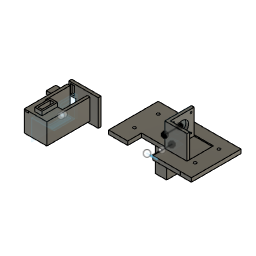
IgracZaBlututSviDelovi v9 (Autodesk Fusion 360 design; units mm, degrees)
Autodesk Fusion 360 part; units mm, degrees
note: some values were not read from the file. Chosen so that the rebuilt part matches the saved one: which bodies a step acts on. Set by a fixed rule: which sketch regions a step uses.
(part 1 of 2)
sketch "Sketch1" plane through (0, 0, 0) normal (0, 0, 1) x (1, 0, 0)
  line L0 (120.0463, 89.9645) -> (140.0463, 89.9645)
  line L1 (140.0463, -0.0355) -> (120.0463, -0.0355)
  line L2 (120.0463, -0.0355) -> (120.0463, 89.9645)
  line L3 (140.0463, 72.4645) -> (140.0463, 69.9645)
  circle A0 centre (140.0463, 69.9645) radius 2.5
  line L4 (140.0463, 69.9645) -> (140.0463, 67.4645)
  line L5 (140.0463, 32.4645) -> (140.0463, 29.9645)
  circle A1 centre (140.0463, 29.9645) radius 2.5
  line L6 (220.0463, 67.4645) -> (220.0463, 69.9645)
  line L7 (220.0463, 32.4645) -> (220.0463, 29.9645)
  circle A2 centre (220.0463, 69.9645) radius 2.5
  circle A3 centre (220.0463, 29.9645) radius 2.5
  line L8 (140.0463, 89.9645) -> (220, 89.9645)
  line L9 (220, 89.9645) -> (240, 89.9645)
  line L10 (240, 89.9645) -> (240, 40)
  line L11 (240, 40) -> (240, 0)
  line L12 (240, 0) -> (140, 0)
  line L13 (180.0463, 29.9645) -> (163.0463, 29.9645)
  line L14 (180.0463, 29.9645) -> (192.0463, 29.9645)
  line L15 (192.0463, 29.9645) -> (192.0463, 6.9645)
  line L16 (192.0463, 6.9645) -> (163.0463, 6.9645)
  line L17 (163.0463, 6.9645) -> (163.0463, 29.9645)
  line L18 (140.0463, 72.4645) -> (140.0463, 67.4645)
  line L19 (140.0463, 32.4645) -> (140.0463, 27.4645)
  line L20 (140.0463, 0) -> (140.0463, -0.0355)
  dimension "d1" = 20
  dimension "d2" = 90
  dimension "d3" = 20
  dimension "d4" = 5
  dimension "d8" = 5
  dimension "d17" = 5
  dimension "d18" = 5
  dimension "d21" = 17
  dimension "d22" = 12
  dimension "d23" = 23
  dimension "d24" = 29
  constraint horizontal L0
  constraint vertical L18
  constraint horizontal L1
  constraint vertical L2
  constraint perpendicular L0 L3
  constraint coincident L3.end A0.centre
  constraint parallel L4 L18
  constraint parallel L5 L18
  constraint coincident L5.end A1.centre
  constraint perpendicular L8 L18
  constraint perpendicular L9 L18
  constraint perpendicular L9 L10
  constraint perpendicular L12 L18
  constraint perpendicular L14 L15
  constraint perpendicular L15 L16
  constraint coincident A1 L5.start
  constraint collinear L18 L19
  constraint coincident A1 L19.end
  constraint coincident L12 L20.start
  constraint collinear L19 L20
  constraint coincident A3 L7.start
  constraint coincident A2 L6.start
  constraint coincident A0 L4.end
  constraint coincident A0 L3.start
  measures "d1" distance of L0.start L0.end
  measures "d2" distance of L0.start L1.end
  measures "d3" distance of L0.end L3.end
  measures "d4" diameter of A0
  measures "d8" diameter of A1
  measures "d17" diameter of A2
  measures "d18" diameter of A3
  measures "d21" distance of L13.start L13.end
  measures "d22" distance of L13.start L14.end
  measures "d23" distance of L14.end L15.end
  measures "d24" distance of L15.end L16.end
extrude "Extrude1" add sketch "Sketch1" along normal blind 7 makes body 1
sketch "Sketch2" plane through (0, 0, 7) normal (0, 0, 1) x (-1, 0, 0)
  circle A0 centre (-220.0463, -69.9645) radius 2.5
  line L0 (-163.0463, -29.9645) -> (-192.0463, -29.9645)
  line L1 (-192.0463, -29.9645) -> (-192.0463, -6.9645)
  line L2 (-192.0463, -6.9645) -> (-163.0463, -6.9645)
  line L3 (-163.0463, -6.9645) -> (-163.0463, -29.9645)
  circle A1 centre (-220.0463, -29.9645) radius 2.5
  circle A2 centre (-140.0463, -29.9645) radius 2.5
  circle A3 centre (-140.0463, -69.9645) radius 2.5
  line L4 (-140.0463, 0) -> (-240, 0)
  line L5 (-240, 0) -> (-240, -89.9645)
  line L6 (-240, -89.9645) -> (-120.0463, -89.9645)
  line L7 (-120.0463, -89.9645) -> (-120.0463, 0.0355)
  line L8 (-120.0463, 0.0355) -> (-140.0463, 0.0355)
  line L9 (-140.0463, 0.0355) -> (-140.0463, 0)
  line L10 (-163.0463, -29.9645) -> (-192.0463, -29.9645)
  line L11 (-192.0463, -29.9645) -> (-192.0463, -6.9645)
  line L12 (-192.0463, -6.9645) -> (-163.0463, -6.9645)
  line L13 (-163.0463, -6.9645) -> (-163.0463, -29.9645)
  constraint horizontal L10
  constraint vertical L11
  constraint horizontal L12
  constraint vertical L13
  constraint coincident L1.end L2.start
  constraint coincident L0.start L3.end
extrude "Extrude2" add sketch "Sketch2" against normal blind 4 contours L0 L1 L2 L3 L10 L11 L12 L13 bodies 1
extrude "Extrude3" add 1 faces at (172.7129, 14.6311, 3) along direction (0, 0, -1) blind 2 on bodies 1 bodies 1
extrude "Extrude4" cut 1 faces at (172.7129, 14.6311, 1) along direction (0, 0, 1) blind 50 on bodies 1 bodies 1
sketch "Sketch3" plane through (0, 0, 0) normal (0, 0, -1) x (1, 0, 0)
  circle A0 centre (220.0463, -69.9645) radius 2.5
  line L0 (192.0463, -29.9645) -> (163.0463, -29.9645)
  line L1 (163.0463, -29.9645) -> (163.0463, -6.9645)
  line L2 (163.0463, -6.9645) -> (192.0463, -6.9645)
  line L3 (192.0463, -6.9645) -> (192.0463, -29.9645)
  circle A1 centre (220.0463, -29.9645) radius 2.5
  circle A2 centre (140.0463, -29.9645) radius 2.5
  circle A3 centre (140.0463, -69.9645) radius 2.5
  line L4 (240, 0) -> (140.0463, 0)
  line L5 (140.0463, 0) -> (140.0463, 0.0355)
  line L6 (140.0463, 0.0355) -> (120.0463, 0.0355)
  line L7 (120.0463, 0.0355) -> (120.0463, -89.9645)
  line L8 (120.0463, -89.9645) -> (240, -89.9645)
  line L9 (240, -89.9645) -> (240, 0)
  line L10 (192.0463, -29.9645) -> (163.0463, -29.9645)
  line L11 (163.0463, -29.9645) -> (163.0463, -6.9645)
  line L12 (163.0463, -6.9645) -> (192.0463, -6.9645)
  line L13 (192.0463, -6.9645) -> (192.0463, -29.9645)
  constraint horizontal L10
  constraint vertical L11
  constraint horizontal L12
  constraint vertical L13
  constraint coincident L1.end L2.start
  constraint coincident L0.start L3.end
extrude "Extrude5" add sketch "Sketch3" against normal blind 4 contours L0 L1 L2 L3 L10 L11 L12 L13 bodies 1
sketch "Sketch4" plane through (0, 0, 0) normal (1, 0, 0) x (0, 1, 0)
sketch "Sketch5" plane through (0, 0, 7) normal (0, 0, 1) x (-1, 0, 0)
  line L0 (-163.0463, -6.9645) -> (-163.0463, -29.9645)
  line L1 (-163.0463, -29.9645) -> (-192.0463, -29.9645)
  line L2 (-192.0463, -29.9645) -> (-192.0463, -6.9645)
  line L3 (-192.0463, -6.9645) -> (-163.0463, -6.9645)
  circle A0 centre (-220.0463, -69.9645) radius 2.5
  circle A1 centre (-220.0463, -29.9645) radius 2.5
  circle A2 centre (-140.0463, -29.9645) radius 2.5
  circle A3 centre (-140.0463, -69.9645) radius 2.5
  line L4 (-140.0463, 0) -> (-240, 0)
  line L5 (-240, 0) -> (-240, -89.9645)
  line L6 (-240, -89.9645) -> (-120.0463, -89.9645)
  line L7 (-120.0463, -89.9645) -> (-120.0463, 0.0355)
  line L8 (-120.0463, 0.0355) -> (-140.0463, 0.0355)
  line L9 (-140.0463, 0.0355) -> (-140.0463, 0)
  line L10 (-50, -90) -> (-86, -90)
  line L11 (-86, -90) -> (-86, -30)
  line L12 (-86, -30) -> (-50, -30)
  line L13 (-50, -30) -> (-50, -90)
  dimension "d35" = 36
  dimension "d37" = 60
  constraint horizontal L10
  constraint vertical L11
  constraint horizontal L12
  constraint vertical L13
  measures "d35" distance of L10.start L10.end
  measures "d37" distance of L10.start L12.end
extrude "Extrude6" add sketch "Sketch5" along normal blind 7 separate body contours L10 L11 L12 L13 makes body 2
sketch "Sketch6" plane through (0, 0, 7) normal (0, 0, -1) x (1, 0, 0)
  line L0 (86, -30) -> (50, -30)
  line L1 (50, -30) -> (50, -90)
  line L2 (50, -90) -> (86, -90)
  line L3 (86, -90) -> (86, -30)
  line L4 (53.231, -87) -> (63, -87)
  line L5 (53.231, -87) -> (53, -87)
  line L6 (53, -87) -> (55, -87)
  line L7 (55, -87) -> (53, -87)
  line L8 (53, -87) -> (53, -78.5331)
  line L9 (53, -78.5331) -> (55, -78.5331)
  line L10 (55, -87) -> (58, -87)
  line L11 (58, -87) -> (63, -87)
  line L12 (63, -87) -> (58, -87)
  line L13 (58, -87) -> (58, -62)
  line L14 (58, -62) -> (63, -62)
  line L15 (63, -62) -> (63, -87)
  line L16 (58, -87) -> (53, -87)
  line L17 (53, -87) -> (53, -62)
  line L18 (53, -62) -> (58, -62)
  line L19 (58, -62) -> (58, -87)
  dimension "d42" = 2
  dimension "d43" = 3
  dimension "d44" = 5
  dimension "d45" = 25
  constraint perpendicular L3 L4
  constraint perpendicular L1 L5
  constraint horizontal L7
  constraint vertical L8
  constraint horizontal L9
  constraint parallel L4 L11
  constraint horizontal L12
  constraint vertical L13
  constraint horizontal L14
  constraint vertical L15
  constraint horizontal L16
  constraint vertical L17
  constraint horizontal L18
  constraint vertical L19
  measures "d42" distance of L6.end L5.end
  measures "d43" distance of L6.end L10.end
  measures "d44" distance of L10.end L4.end
  measures "d45" distance of L4.end L14.end
extrude "Extrude7" add sketch "Sketch6" along normal blind 7 contours L4 L5 L6 L7 L8 L10 L13 L16 L17 L18 L19 | L4 L11 L12 L13 L14 L15 L19 bodies 2
sketch "Sketch7" plane through (0, 0, 7) normal (0, 0, -1) x (1, 0, 0)
  line L0 (63, -62) -> (63, -87)
  line L1 (63, -87) -> (53, -87)
  line L2 (53, -87) -> (53, -62)
  line L3 (53, -62) -> (63, -62)
  line L4 (86, -30) -> (50, -30)
  line L5 (50, -30) -> (50, -90)
  line L6 (50, -90) -> (86, -90)
  line L7 (86, -90) -> (86, -30)
  line L8 (53, -87) -> (71, -87)
  line L9 (71, -87) -> (86, -87)
  line L10 (86, -87) -> (83, -87)
  line L11 (83, -87) -> (73, -87)
  line L12 (73, -87) -> (73, -62)
  line L13 (73, -62) -> (83, -62)
  line L14 (83, -62) -> (83, -87)
  dimension "d48" = 3
  dimension "d49" = 10
  dimension "d50" = 25
  constraint coincident L1.end L2.start
  constraint coincident L7 L9.end
  constraint perpendicular L7 L9
  constraint perpendicular L7 L10
  constraint horizontal L11
  constraint vertical L12
  constraint horizontal L13
  constraint vertical L14
  measures "d48" distance of L9.end L10.end
  measures "d49" distance of L10.end L11.end
  measures "d50" distance of L10.end L13.end
extrude "Extrude8" add sketch "Sketch7" along normal blind 7 contours L9 L11 L12 L13 L14 bodies 2
extrude "Extrude9" cut 1 faces at (59.6667, 75.8444, 0) along direction (0, 0, 1) blind 7 on bodies 2 bodies 2
sketch "Sketch8" plane through (73, 0, 0) normal (-1, 0, 0) x (0, -1, 0)
  line L0 (-62, 7) -> (-87, 7)
  line L1 (-87, 7) -> (-87, 0)
  line L2 (-87, 0) -> (-62, 0)
  line L3 (-62, 0) -> (-62, 7)
  line L4 (-87, 0) -> (-84.5, 0)
  line L5 (-84.5, 0) -> (-84.5, 7)
  line L6 (-62, 0) -> (-64.5, 0)
  line L7 (-64.5, 0) -> (-64.5, 7)
  line L8 (-74.5, 0) -> (-74.5, 2)
  line L9 (-74.5, 2) -> (-84.5, 2)
  line L10 (-64.5, 2) -> (-74.5, 2)
  line L11 (-64.5, 2) -> (-64.5, 9)
  dimension "d55" = 2.5
  dimension "d56" = 2.5
  dimension "d57" = 2
  dimension "d58" = 7
  constraint coincident L1.end L2.start
  constraint perpendicular L1 L4
  constraint coincident L0 L5.end
  constraint perpendicular L0 L5
  constraint coincident L2.end L3.start
  constraint perpendicular L3 L6
  constraint coincident L0 L7.end
  constraint perpendicular L0 L7
  constraint midpoint L2 L8.start
  constraint perpendicular L2 L8
  constraint coincident L5 L9.end
  constraint perpendicular L5 L9
  constraint coincident L7 L10.start
  constraint perpendicular L7 L10
  constraint perpendicular L10 L11
  measures "d55" distance of L1.end L4.end
  measures "d56" distance of L2.end L6.end
  measures "d57" distance of L8.start L8.end
  measures "d58" distance of L10.start L11.end
extrude "Extrude10" cut sketch "Sketch8" against normal blind 5 contours L0 L5 L7 L9 L10 L11 bodies 2
extrude "Extrude11" cut 1 faces at (69.6667, 40.6667, 7) along direction (0, 0, 1) blind 2 on bodies 2 bodies 2
extrude "Extrude12" add 1 faces at (62, 70, 14) along direction (0, 0, 1) blind 2 on bodies 2 bodies 2
sketch "Sketch9" plane through (78, 0, 0) normal (-1, 0, 0) x (0, -1, 0)
  line L0 (-84.5, 2) -> (-64.5, 2)
  line L1 (-64.5, 2) -> (-64.5, 9)
  line L2 (-64.5, 9) -> (-84.5, 9)
  line L3 (-84.5, 9) -> (-84.5, 2)
  line L4 (-69.5871, 9) -> (-69.5871, 7)
  line L5 (-69.5871, 7) -> (-64.5, 7)
  line L6 (-69.5871, 7) -> (-84.5, 7)
  constraint coincident L2 L4.start
  constraint perpendicular L2 L4
  constraint coincident L1 L5.end
  constraint perpendicular L1 L5
  constraint coincident L3 L6.end
  constraint perpendicular L3 L6
extrude "Extrude13" add sketch "Sketch9" along normal blind 5 contours L2 L3 L4 L6 | L1 L2 L4 L5 bodies 2
move_body "Move1" bodies 2 to x (-1, 0, 0) y (0, 1, 0) z (0, 0, -1) at (136, 10, 16)
sketch "Sketch10" plane through (0, 0, 0) normal (0, 0, -1) x (1, 0, 0)
  circle A0 centre (220.0463, -69.9645) radius 2.5
  circle A1 centre (220.0463, -29.9645) radius 2.5
  circle A2 centre (140.0463, -29.9645) radius 2.5
  circle A3 centre (140.0463, -69.9645) radius 2.5
  line L0 (240, 0) -> (140.0463, 0)
  line L1 (140.0463, 0) -> (140.0463, 0.0355)
  line L2 (140.0463, 0.0355) -> (120.0463, 0.0355)
  line L3 (120.0463, 0.0355) -> (120.0463, -89.9645)
  line L4 (120.0463, -89.9645) -> (240, -89.9645)
  line L5 (240, -89.9645) -> (240, 0)
  circle A4 centre (140.0463, -29.9645) radius 7.5
  circle A5 centre (140.0463, -69.9645) radius 7.5
  circle A6 centre (220.0463, -69.9645) radius 7.5
  circle A7 centre (220.0463, -29.9645) radius 7.5
  dimension "d67" = 15
  dimension "d68" = 15
  dimension "d69" = 15
  dimension "d70" = 15
  constraint concentric A2 A4
  constraint concentric A3 A5
  constraint concentric A0 A6
  constraint concentric A1 A7
  measures "d67" diameter of A4
  measures "d68" diameter of A5
  measures "d69" diameter of A6
  measures "d70" diameter of A7
extrude "Extrude14" add sketch "Sketch10" along normal blind 15 contours A4 | A5 | A6 | A7 bodies 1
sketch "Sketch11" plane through (0, 0, 0) normal (0, 0, -1) x (1, 0, 0)
  circle A0 centre (140.0463, -69.9645) radius 7.5
  circle A1 centre (220.0463, -69.9645) radius 7.5
  circle A2 centre (140.0463, -29.9645) radius 7.5
  circle A3 centre (220.0463, -29.9645) radius 7.5
  line L0 (240, 0) -> (140.0463, 0)
  line L1 (140.0463, 0) -> (140.0463, 0.0355)
  line L2 (140.0463, 0.0355) -> (120.0463, 0.0355)
  line L3 (120.0463, 0.0355) -> (120.0463, -89.9645)
  line L4 (120.0463, -89.9645) -> (240, -89.9645)
  line L5 (240, -89.9645) -> (240, 0)
move_body "Move2" bodies 1 to x (-1, 0, 0) y (0, 1, 0) z (0, 0, -1) at (340.3336, 0, 7.2628)
extrude "Extrude15" cut 1 faces at (59.6667, 87.8333, 9) along direction (0, 0, -1) blind 1 on bodies 2 bodies 2
extrude "Extrude16" cut 1 faces at (114.4912, 70.4613, 22.2628) along direction (0, 0, -1) blind 15 on bodies 1 bodies 1
extrude "Extrude17" add 1 faces at (114.4819, 30.3371, 22.2628) along direction (0, 0, 1) blind 15 on bodies 1 bodies 1
extrude "Extrude18" cut 1 faces at (114.4819, 30.3371, 37.2628) along direction (0, 0, -1) blind 30 on bodies 1 bodies 1
extrude "Extrude19" cut 1 faces at (194.4819, 30.3371, 22.2628) along direction (0, 0, -1) blind 15 on bodies 1 bodies 1
extrude "Extrude20" cut 1 faces at (194.4912, 70.4613, 22.2628) along direction (0, 0, -1) blind 15 on bodies 1 bodies 1
sketch "Sketch12" plane through (0, 0, 7.2628) normal (0, 0, 1) x (-1, 0, 0)
  circle A0 centre (-200.2873, -69.9645) radius 2.5
  circle A1 centre (-200.2873, -29.9645) radius 2.5
  circle A2 centre (-120.2873, -29.9645) radius 2.5
  circle A3 centre (-120.2873, -69.9645) radius 2.5
  line L0 (-100.3336, 0) -> (-200.2873, 0)
  line L1 (-200.2873, 0) -> (-200.2873, 0.0355)
  line L2 (-200.2873, 0.0355) -> (-220.2873, 0.0355)
  line L3 (-220.2873, 0.0355) -> (-220.2873, -89.9645)
  line L4 (-220.2873, -89.9645) -> (-100.3336, -89.9645)
  line L5 (-100.3336, -89.9645) -> (-100.3336, 0)
  line L6 (-120.2873, -29.9645) -> (-120.2873, -69.9645)
  constraint coincident A2.centre L6.start
  constraint coincident A3.centre L6.end
extrude "Extrude21" add sketch "Sketch12" against normal blind 7 contours A2 bodies 1
sketch "Sketch13" plane through (0, 0, 7.2628) normal (0, 0, 1) x (-1, 0, 0)
  circle A0 centre (-200.2873, -69.9645) radius 2.5
  circle A1 centre (-200.2873, -29.9645) radius 2.5
  circle A2 centre (-120.2873, -69.9645) radius 2.5
  line L0 (-100.3336, 0) -> (-200.2873, 0)
  line L1 (-200.2873, 0) -> (-200.2873, 0.0355)
  line L2 (-200.2873, 0.0355) -> (-220.2873, 0.0355)
  line L3 (-220.2873, 0.0355) -> (-220.2873, -89.9645)
  line L4 (-220.2873, -89.9645) -> (-100.3336, -89.9645)
  line L5 (-100.3336, -89.9645) -> (-100.3336, 0)
extrude "Extrude22" add sketch "Sketch13" against normal blind 7 contours A1 bodies 1
sketch "Sketch14" plane through (0, 0, 7.2628) normal (0, 0, 1) x (-1, 0, 0)
  circle A0 centre (-200.2873, -69.9645) radius 2.5
  circle A1 centre (-120.2873, -69.9645) radius 2.5
  line L0 (-100.3336, 0) -> (-200.2873, 0)
  line L1 (-200.2873, 0) -> (-200.2873, 0.0355)
  line L2 (-200.2873, 0.0355) -> (-220.2873, 0.0355)
  line L3 (-220.2873, 0.0355) -> (-220.2873, -89.9645)
  line L4 (-220.2873, -89.9645) -> (-100.3336, -89.9645)
  line L5 (-100.3336, -89.9645) -> (-100.3336, 0)
  line L6 (-120.2873, -69.9645) -> (-120.2873, -26.9645)
  circle A2 centre (-120.2873, -26.9645) radius 2.5
  line L7 (-200.2873, -69.9645) -> (-200.2873, -24.9645)
  circle A3 centre (-200.2873, -24.9645) radius 2.5
  dimension "d89" = 43
  dimension "d90" = 5
  dimension "d91" = 45
  dimension "d92" = 5
  constraint coincident A1.centre L6.start
  constraint vertical L6
  constraint coincident L6.end A2.centre
  constraint coincident A0.centre L7.start
  constraint vertical L7
  constraint coincident L7.end A3.centre
  measures "d89" distance of A1.centre L6.end
  measures "d90" diameter of A2
  measures "d91" distance of A0.centre L7.end
  measures "d92" diameter of A3
extrude "Extrude23" cut sketch "Sketch14" against normal blind 10 contours A2 | A3 bodies 1
sketch "Sketch15" plane through (0, 0, 7.2628) normal (0, 0, 1) x (-1, 0, 0)
  circle A0 centre (-200.2873, -24.9645) radius 2.5
  circle A1 centre (-120.2873, -26.9645) radius 2.5
  circle A2 centre (-200.2873, -69.9645) radius 2.5
  circle A3 centre (-120.2873, -69.9645) radius 2.5
  line L0 (-100.3336, 0) -> (-200.2873, 0)
  line L1 (-200.2873, 0) -> (-200.2873, 0.0355)
  line L2 (-200.2873, 0.0355) -> (-220.2873, 0.0355)
  line L3 (-220.2873, 0.0355) -> (-220.2873, -89.9645)
  line L4 (-220.2873, -89.9645) -> (-100.3336, -89.9645)
  line L5 (-100.3336, -89.9645) -> (-100.3336, 0)
extrude "Extrude24" add sketch "Sketch15" against normal blind 7 contours A0 bodies 1
sketch "Sketch16" plane through (0, 0, 7.2628) normal (0, 0, 1) x (-1, 0, 0)
  circle A0 centre (-120.2873, -26.9645) radius 2.5
  circle A1 centre (-200.2873, -69.9645) radius 2.5
  circle A2 centre (-120.2873, -69.9645) radius 2.5
  line L0 (-100.3336, 0) -> (-200.2873, 0)
  line L1 (-200.2873, 0) -> (-200.2873, 0.0355)
  line L2 (-200.2873, 0.0355) -> (-220.2873, 0.0355)
  line L3 (-220.2873, 0.0355) -> (-220.2873, -89.9645)
  line L4 (-220.2873, -89.9645) -> (-100.3336, -89.9645)
  line L5 (-100.3336, -89.9645) -> (-100.3336, 0)
  line L6 (-200.2873, -69.9645) -> (-200.2873, -26.9645)
  circle A3 centre (-200.2873, -26.9645) radius 2.5
  dimension "d97" = 43
  dimension "d98" = 5
  constraint coincident A1.centre L6.start
  constraint vertical L6
  constraint coincident L6.end A3.centre
  measures "d97" distance of A1.centre L6.end
  measures "d98" diameter of A3
extrude "Extrude25" cut sketch "Sketch16" against normal blind 10 contours A3 bodies 1
sketch "Sketch17" plane through (0, 0, 7.2628) normal (0, 0, 1) x (-1, 0, 0)
  circle A0 centre (-200.2873, -26.9645) radius 2.5
  circle A1 centre (-120.2873, -26.9645) radius 2.5
  circle A2 centre (-200.2873, -69.9645) radius 2.5
  circle A3 centre (-120.2873, -69.9645) radius 2.5
  line L0 (-100.3336, 0) -> (-200.2873, 0)
  line L1 (-200.2873, 0) -> (-200.2873, 0.0355)
  line L2 (-200.2873, 0.0355) -> (-220.2873, 0.0355)
  line L3 (-220.2873, 0.0355) -> (-220.2873, -89.9645)
  line L4 (-220.2873, -89.9645) -> (-100.3336, -89.9645)
  line L5 (-100.3336, -89.9645) -> (-100.3336, 0)
  line L6 (-200.2873, -26.9645) -> (-120.2873, -26.9645)
  line L7 (-120.2873, -26.9645) -> (-120.2873, -69.9645)
  line L8 (-120.2873, -69.9645) -> (-200.2873, -69.9645)
  line L9 (-200.2873, -69.9645) -> (-200.2873, -26.9645)
  line L10 (-200.2873, -26.9645) -> (-120.2873, -26.9645)
  line L11 (-120.2873, -26.9645) -> (-160.2873, -26.9645)
  line L12 (-160.2873, -26.9645) -> (-160.2873, -69.9645)
  line L13 (-160.2873, -26.9645) -> (-190.2873, -26.9645)
  line L14 (-190.2873, -26.9645) -> (-190.2873, -69.9645)
  line L15 (-190.2873, -26.9645) -> (-155.2873, -26.9645)
  line L16 (-155.2873, -26.9645) -> (-155.2873, -69.9645)
  line L17 (-155.2873, -69.9645) -> (-190.2873, -69.9645)
  dimension "d101" = 40
  dimension "d102" = 30
  dimension "d103" = 35
  constraint coincident A0.centre L6.start
  constraint coincident A1.centre L6.end
  constraint coincident A3.centre L7.end
  constraint coincident A2.centre L8.end
  constraint parallel L10 L11
  constraint midpoint L8 L12.end
  constraint perpendicular L12 L13
  constraint coincident L8 L14.end
  constraint perpendicular L8 L14
  constraint perpendicular L12 L15
  constraint coincident L8 L16.end
  constraint perpendicular L8 L16
  measures "d101" distance of A1.centre L11.end
  measures "d102" distance of L11.end L13.end
  measures "d103" distance of L13.end L15.end
extrude "Extrude26" cut sketch "Sketch17" against normal blind 2 contours L6 L8 L10 L12 L13 L14 L15 L17 | L6 L8 L10 L11 L12 L15 L16 L17 bodies 1
sketch "Sketch18" plane through (0, 0, 7.2628) normal (0, 0, 1) x (-1, 0, 0)
  line L0 (-155.2873, -69.9645) -> (-190.2873, -69.9645)
  line L1 (-190.2873, -69.9645) -> (-190.2873, -26.9645)
  line L2 (-190.2873, -26.9645) -> (-155.2873, -26.9645)
  line L3 (-155.2873, -26.9645) -> (-155.2873, -69.9645)
  circle A0 centre (-200.2873, -26.9645) radius 2.5
  circle A1 centre (-120.2873, -26.9645) radius 2.5
  circle A2 centre (-200.2873, -69.9645) radius 2.5
  circle A3 centre (-120.2873, -69.9645) radius 2.5
  line L4 (-100.3336, 0) -> (-200.2873, 0)
  line L5 (-200.2873, 0) -> (-200.2873, 0.0355)
  line L6 (-200.2873, 0.0355) -> (-220.2873, 0.0355)
  line L7 (-220.2873, 0.0355) -> (-220.2873, -89.9645)
  line L8 (-220.2873, -89.9645) -> (-100.3336, -89.9645)
  line L9 (-100.3336, -89.9645) -> (-100.3336, 0)
  line L10 (-155.2873, -26.9645) -> (-155.2873, -48.4645)
  line L11 (-155.2873, -48.4645) -> (-150.2873, -48.4645)
  line L12 (-150.2873, -48.4645) -> (-150.2873, -26.9645)
  line L13 (-150.2873, -26.9645) -> (-150.2873, -21.9645)
  line L14 (-150.2873, -21.9645) -> (-190.2873, -21.9645)
  line L15 (-190.2873, -21.9645) -> (-190.2873, -26.9645)
  line L16 (-150.2873, -48.4645) -> (-150.2873, -69.9645)
  line L17 (-150.2873, -69.9645) -> (-155.2873, -69.9645)
  dimension "d106" = 21.5
  dimension "d107" = 5
  dimension "d108" = 21.5
  dimension "d109" = 5
  dimension "d110" = 21.5
  constraint coincident L2.end L3.start
  constraint perpendicular L2 L10
  constraint perpendicular L3 L11
  constraint perpendicular L11 L12
  constraint parallel L12 L13
  constraint perpendicular L13 L14
  constraint coincident L1.end L2.start
  constraint perpendicular L2 L15
  constraint perpendicular L11 L16
  constraint coincident L0.start L3.end
  measures "d106" distance of L2.end L10.end
  measures "d107" distance of L10.end L11.end
  measures "d108" distance of L11.end L12.end
  measures "d109" distance of L12.end L13.end
  measures "d110" distance of L11.end L16.end
extrude "Extrude27" add sketch "Sketch18" along normal blind 43.2 contours L3 L11 L16 L17 | L2 L3 L10 L11 L12 L13 L14 L15 bodies 1
sketch "Sketch19" plane through (150.2873, 0, 0) normal (-1, 0, 0) x (0, -1, 0)
  line L0 (-69.9645, 7.2628) -> (-21.9645, 7.2628)
  line L1 (-21.9645, 7.2628) -> (-21.9645, 50.4628)
  line L2 (-21.9645, 50.4628) -> (-69.9645, 50.4628)
  line L3 (-69.9645, 50.4628) -> (-69.9645, 7.2628)
  line L4 (-69.9645, 50.4628) -> (-64.3645, 50.4628)
  line L5 (-69.9645, 50.4628) -> (-69.9645, 44.8628)
  line L6 (-69.9645, 44.8628) -> (-64.3645, 44.8628)
  circle A0 centre (-64.3645, 44.8628) radius 1.5
  line L7 (-21.9645, 50.4628) -> (-32.5645, 50.4628)
  line L8 (-21.9645, 50.4628) -> (-21.9645, 44.8628)
  line L9 (-21.9645, 44.8628) -> (-69.9645, 44.8628)
  line L10 (-69.9645, 7.2628) -> (-64.3645, 7.2628)
  line L11 (-64.3645, 7.2628) -> (-64.3645, 50.4628)
  line L12 (-69.9645, 7.2628) -> (-69.9645, 12.8628)
  line L13 (-69.9645, 12.8628) -> (-21.9645, 12.8628)
  line L14 (-21.9645, 7.2628) -> (-21.9645, 50.4628)
  line L15 (-32.5645, 50.4628) -> (-32.5645, 7.2628)
  circle A1 centre (-32.5645, 44.8628) radius 1.5
  circle A2 centre (-32.5645, 12.8628) radius 1.5
  circle A3 centre (-64.3645, 12.8628) radius 1.5
  dimension "d113" = 5.6
  dimension "d114" = 5.6
  dimension "d115" = 5.6
  dimension "d116" = 3
  dimension "d117" = 10.6
  dimension "d118" = 5.6
  dimension "d119" = 5.6
  dimension "d120" = 5.6
  dimension "d121" = 3
  dimension "d122" = 3
  dimension "d123" = 3
  constraint coincident L2.end L3.start
  constraint perpendicular L3 L4
  constraint perpendicular L4 L5
  constraint perpendicular L3 L6
  constraint coincident L6.end A0.centre
  constraint coincident L1.end L2.start
  constraint perpendicular L1 L7
  constraint perpendicular L7 L8
  constraint coincident L0.start L3.end
  constraint perpendicular L3 L10
  constraint perpendicular L10 L12
  constraint coincident L1 L13.end
  constraint perpendicular L1 L13
  constraint coincident L0.end L1.start
  constraint coincident L0 L15.end
  constraint perpendicular L0 L15
  constraint coincident L9 A1.centre
  constraint coincident L15 A1.centre
  constraint coincident L13 A2.centre
  constraint coincident L15 A2.centre
  constraint coincident L13 A3.centre
  constraint coincident L11 A3.centre
  measures "d113" distance of L2.end L4.end
  measures "d114" distance of L2.end L5.end
  measures "d115" distance of L5.end L6.end
  measures "d116" diameter of A0
  measures "d117" distance of L1.end L7.end
  measures "d118" distance of L1.end L8.end
  measures "d119" distance of L0.start L10.end
  measures "d120" distance of L0.start L12.end
  measures "d121" diameter of A1
  measures "d122" diameter of A2
  measures "d123" diameter of A3
extrude "Extrude28" cut sketch "Sketch19" against normal blind 60 contours L11 L13 A3 | L11 L13 A3 | L11 L13 A3 | L13 L15 A2 | L13 L15 A2 | L11 L13 A3 | L6 A0 L9 L11 | L6 A0 L9 L11 | L13 L15 A2 | L13 L15 A2 | A0 L9 L11 | A0 L9 L11 | L9 L15 A1 | L9 L15 A1 | L9 L15 A1 | L9 L15 A1 bodies 1
sketch "Sketch20" plane through (150.2873, 0, 0) normal (-1, 0, 0) x (0, -1, 0)
  circle A0 centre (-32.5645, 44.8628) radius 1.5
  circle A1 centre (-32.5645, 12.8628) radius 1.5
  circle A2 centre (-64.3645, 44.8628) radius 1.5
  circle A3 centre (-64.3645, 12.8628) radius 1.5
  line L0 (-69.9645, 7.2628) -> (-21.9645, 7.2628)
  line L1 (-21.9645, 7.2628) -> (-21.9645, 50.4628)
  line L2 (-21.9645, 50.4628) -> (-69.9645, 50.4628)
  line L3 (-69.9645, 50.4628) -> (-69.9645, 7.2628)
  line L4 (-69.9645, 50.4628) -> (-48.4645, 50.4628)
  line L5 (-48.4645, 50.4628) -> (-48.4645, 28.8628)
  circle A4 centre (-48.4645, 28.8628) radius 11.5
  dimension "d126" = 21.5
  dimension "d127" = 21.6
  dimension "d128" = 23
  constraint coincident L2.end L3.start
  constraint perpendicular L3 L4
  constraint perpendicular L4 L5
  constraint coincident L5.end A4.centre
  measures "d126" distance of L2.end L4.end
  measures "d127" distance of L4.end L5.end
  measures "d128" diameter of A4
extrude "Extrude29" cut sketch "Sketch20" against normal blind 50 contours A4 bodies 1
sketch "Sketch21" plane through (0, 0, 7.2628) normal (0, 0, 1) x (-1, 0, 0)
  line L0 (-100.3336, 0) -> (-200.2873, 0)
  line L1 (-200.2873, 0) -> (-200.2873, 0.0355)
  line L2 (-200.2873, 0.0355) -> (-220.2873, 0.0355)
  line L3 (-220.2873, 0.0355) -> (-220.2873, -89.9645)
  line L4 (-220.2873, -89.9645) -> (-100.3336, -89.9645)
  line L5 (-100.3336, -89.9645) -> (-100.3336, 0)
  circle A0 centre (-120.2873, -69.9645) radius 2.5
  circle A1 centre (-200.2873, -69.9645) radius 2.5
  circle A2 centre (-120.2873, -26.9645) radius 2.5
  circle A3 centre (-200.2873, -26.9645) radius 2.5
  line L6 (-190.2873, -26.9645) -> (-190.2873, -21.9645)
  line L7 (-190.2873, -21.9645) -> (-150.2873, -21.9645)
  line L8 (-150.2873, -21.9645) -> (-150.2873, -69.9645)
  line L9 (-150.2873, -69.9645) -> (-155.2873, -69.9645)
  line L10 (-155.2873, -69.9645) -> (-190.2873, -69.9645)
  line L11 (-190.2873, -69.9645) -> (-190.2873, -26.9645)
sketch "Sketch22" plane through (0, 0, 0.2628) normal (0, 0, -1) x (1, 0, 0)
  circle A0 centre (200.2873, -26.9645) radius 2.5
  circle A1 centre (120.2873, -26.9645) radius 2.5
  line L0 (177.2873, -6.9645) -> (177.2873, -29.9645)
  line L1 (177.2873, -29.9645) -> (148.2873, -29.9645)
  line L2 (148.2873, -29.9645) -> (148.2873, -6.9645)
  line L3 (148.2873, -6.9645) -> (177.2873, -6.9645)
  circle A2 centre (120.2873, -69.9645) radius 2.5
  circle A3 centre (200.2873, -69.9645) radius 2.5
  line L4 (200.2873, 0) -> (100.3336, 0)
  line L5 (100.3336, 0) -> (100.3336, -89.9645)
  line L6 (100.3336, -89.9645) -> (220.2873, -89.9645)
  line L7 (220.2873, -89.9645) -> (220.2873, 0.0355)
  line L8 (220.2873, 0.0355) -> (200.2873, 0.0355)
  line L9 (200.2873, 0.0355) -> (200.2873, 0)
  line L10 (120.2873, -69.9645) -> (120.2873, -48.4645)
  line L11 (120.2873, -48.4645) -> (200.2873, -48.4645)
  dimension "d131" = 21.5
  dimension "d132" = 80
  constraint coincident A2.centre L10.start
  constraint parallel L5 L10
  constraint perpendicular L10 L11
  measures "d131" distance of A2.centre L10.end
  measures "d132" distance of L10.end L11.end
extrude "Extrude30" add sketch "Sketch22" along normal blind 3 separate body contours L0 L1 L2 L3 makes body 3
extrude "Extrude31" cut 1 faces at (157.954, 14.6311, -2.7372) along direction (0, 0, 1) blind 1 on bodies 3 bodies 3
extrude "Extrude32" cut 1 faces at (157.954, 14.6311, -1.7372) along direction (0, 0, 1) blind 1 on bodies 3 bodies 3
extrude "Extrude33" cut 1 faces at (157.954, 14.6311, -0.7372) along direction (0, 0, 1) blind 1 on bodies 3 bodies 3
extrude "Extrude34" add 1 faces at (167.6206, 22.2978, 3.2628) along direction (0, 0, -1) blind 3 on bodies 1 bodies 2 1
sketch "Sketch23" plane through (0, 0, 0.2628) normal (0, 0, -1) x (1, 0, 0)
  circle A0 centre (200.2873, -26.9645) radius 2.5
  circle A1 centre (120.2873, -26.9645) radius 2.5
  circle A2 centre (120.2873, -69.9645) radius 2.5
  circle A3 centre (200.2873, -69.9645) radius 2.5
  line L0 (200.2873, 0) -> (100.3336, 0)
  line L1 (100.3336, 0) -> (100.3336, -89.9645)
  line L2 (100.3336, -89.9645) -> (220.2873, -89.9645)
  line L3 (220.2873, -89.9645) -> (220.2873, 0.0355)
  line L4 (220.2873, 0.0355) -> (200.2873, 0.0355)
  line L5 (200.2873, 0.0355) -> (200.2873, 0)
  line L6 (120.2873, -69.9645) -> (120.2873, -48.4645)
  line L7 (200.2873, -69.9645) -> (200.2873, -26.9645)
  line L8 (200.2873, -26.9645) -> (200.2873, -48.4645)
  line L9 (200.2873, -48.4645) -> (160.2873, -48.4645)
  line L10 (160.2873, -48.4645) -> (155.2873, -48.4645)
  line L11 (155.2873, -48.4645) -> (155.2873, -70)
  line L12 (155.2873, -70) -> (155.2873, -48.4645)
  line L13 (155.2873, -48.4645) -> (155.2873, -30)
  line L14 (155.2873, -48.4645) -> (150, -48.4645)
  line L15 (155.2873, -48.4645) -> (150.2873, -48.4645)
  line L16 (150, -70) -> (150, -30)
  line L17 (150, -30) -> (150.3104, 0)
  line L18 (200.2873, -48.4645) -> (200.2873, -42.7621)
  line L19 (200.2873, -48.4645) -> (200.2873, -38.4645)
  line L20 (120.2873, -38.4645) -> (120.2873, -58.4645)
  line L21 (150, -48.4645) -> (150, -59.8645)
  line L22 (130, -59.8645) -> (142.4, -59.8645)
  line L23 (130, -59.8645) -> (130, -37.0645)
  line L24 (130, -37.0645) -> (142.4, -37.0645)
  line L25 (142.4, -59.8645) -> (142.4, -37.0645)
  line L26 (120.2873, -58.4645) -> (126, -58.4645)
  line L27 (146.4, -58.4645) -> (200.2873, -58.4645)
  line L28 (120.2873, -48.4645) -> (126, -48.4645)
  line L29 (146.4, -48.4645) -> (160.2873, -48.4645)
  line L30 (200.2873, -38.4645) -> (146.4, -38.4645)
  line L31 (126, -38.4645) -> (120.2873, -38.4645)
  line L32 (150.2873, -48.4645) -> (146.4, -48.4243)
  line L33 (130, -67.8645) -> (142.4, -67.8645)
  line L34 (130, -29.0645) -> (142.4, -29.0645)
  line L35 (130, -29.0645) -> (126, -29.0645)
  line L36 (126, -29.0645) -> (126, -60)
  line L37 (126, -60) -> (126, -68)
  line L38 (142.4, -67.8645) -> (146.4, -67.8645)
  line L39 (146.4, -67.8645) -> (146.4, -35)
  line L40 (146.4, -35) -> (146.4, -29)
  line L41 (146.4, -29) -> (142.4, -29.0645)
  line L42 (126, -68) -> (130, -67.8645)
  line L43 (128.2885, -29.0645) -> (128.2885, 0)
  line L44 (150, -59.8645) -> (146.4, -59.8645)
  line L45 (142.4, -59.8645) -> (130, -59.8645)
  dimension "d143" = 21.5
  dimension "d144" = 40
  dimension "d145" = 5
  dimension "d146" = 5
  dimension "d148" = 10
  dimension "d149" = 80
  dimension "d150" = 20
  dimension "d151" = 11.4
  dimension "d152" = 20
  dimension "d153" = 12.4
  dimension "d154" = 22.8
  dimension "d155" = 12.4
  dimension "d156" = 8
  dimension "d157" = 12.4
  dimension "d158" = 8
  dimension "d159" = 12.4
  dimension "d160" = 4
  dimension "d161" = 4
  constraint coincident A2.centre L6.start
  constraint vertical L6
  constraint perpendicular L6 L28
  constraint coincident A3.centre L7.start
  constraint coincident A0.centre L7.end
  constraint midpoint L7 L8.end
  constraint perpendicular L7 L10
  constraint perpendicular L11 L28
  constraint perpendicular L13 L28
  constraint coincident L14.end L28
  constraint perpendicular L11 L15
  constraint perpendicular L16 L28
  constraint midpoint L0 L17.end
  constraint perpendicular L17 L32
  constraint coincident L0 L43.end
  constraint coincident L8 L18.end
  constraint perpendicular L9 L18
  constraint perpendicular L9 L19
  constraint perpendicular L13 L30
  constraint perpendicular L20 L30
  constraint coincident L7 L27.end
  constraint perpendicular L7 L26
  constraint perpendicular L21 L28
  constraint perpendicular L16 L44
  constraint parallel L22 L44
  constraint perpendicular L23 L30
  constraint perpendicular L23 L24
  constraint collinear L26 L27
  constraint collinear L28 L29
  constraint collinear L30 L31
  constraint perpendicular L26 L36
  constraint parallel L36 L37
  constraint perpendicular L30 L39
  constraint parallel L39 L40
  constraint coincident L39 L30.end
  constraint coincident L39 L29.start
  constraint coincident L35 L43.start
  constraint coincident L36 L31.start
  constraint coincident L39 L32.end
  constraint coincident L39 L27.start
  constraint coincident L39 L44.end
  constraint collinear L44 L45
  constraint coincident L36 L26.end
  constraint coincident L36 L28.end
  measures "d143" distance of A2.centre L6.end
  measures "d144" distance of L6.end L9.end
  measures "d145" distance of L9.end L10.end
  measures "d146" distance of L10.end L15.end
  measures "d148" distance of L8.end L19.end
  measures "d149" distance of L19.end L20.start
  measures "d150" distance of L20.start L20.end
  measures "d151" distance of L14.end L21.end
  measures "d152" distance of L21.end L22.start
  measures "d153" distance of L22.start L22.end
  measures "d154" distance of L22.start L23.end
  measures "d155" distance of L23.end L24.end
  measures "d156" distance of L22.start L33.start
  measures "d157" distance of L33.start L33.end
  measures "d158" distance of L23.end L34.start
  measures "d159" distance of L34.start L34.end
  measures "d160" distance of L34.start L35.end
  measures "d161" distance of L33.end L38.end
extrude "Extrude35" add sketch "Sketch23" along normal blind 45 contours L33 L34 L35 L36 L37 L38 L39 L40 L41 L42 bodies 1
sketch "Sketch24" plane through (146.4, 0, 0) normal (1, 0, 0) x (0, 1, 0)
  line L0 (67.8645, 0.2628) -> (29, 0.2628)
  line L1 (29, 0.2628) -> (29, -44.7372)
  line L2 (29, -44.7372) -> (67.8645, -44.7372)
  line L3 (67.8645, -44.7372) -> (67.8645, 0.2628)
  line L4 (67.8645, 0.2628) -> (48.3645, 0.2628)
  line L5 (48.3645, 0.2628) -> (48.3645, -6.7372)
  line L6 (48.3645, -6.7372) -> (37.3645, -6.7372)
  line L7 (48.3645, -6.7372) -> (59.3645, -6.7372)
  line L8 (37.3645, -6.7372) -> (37.3645, -28.7372)
  line L9 (37.3645, -28.7372) -> (59.3645, -28.7372)
  line L10 (59.3645, -28.7372) -> (59.3645, -6.7372)
  dimension "d164" = 19.5
  dimension "d165" = 7
  dimension "d166" = 11
  dimension "d167" = 11
  dimension "d168" = 22
  dimension "d169" = 22
  constraint coincident L0.start L3.end
  constraint perpendicular L3 L4
  constraint perpendicular L4 L5
  constraint perpendicular L5 L6
  constraint perpendicular L5 L7
  constraint perpendicular L6 L8
  constraint perpendicular L8 L9
  measures "d164" distance of L0.start L4.end
  measures "d165" distance of L4.end L5.end
  measures "d166" distance of L5.end L6.end
  measures "d167" distance of L5.end L7.end
  measures "d168" distance of L6.end L8.end
  measures "d169" distance of L8.end L9.end
extrude "Extrude36" cut sketch "Sketch24" against normal blind 50 contours L6 L7 L8 L9 L10 bodies 1
extrude "Extrude37" add 1 faces at (139.6, 65.1978, -44.7372) along direction (0, 0, -1) blind 3 on bodies 1 bodies 1
sketch "Sketch25" plane through (0, 0, -47.7372) normal (0, 0, -1) x (1, 0, 0)
  line L0 (142.4, -37.0645) -> (142.4, -59.8645)
  line L1 (142.4, -59.8645) -> (130, -59.8645)
  line L2 (130, -59.8645) -> (130, -37.0645)
  line L3 (130, -37.0645) -> (142.4, -37.0645)
  line L4 (142.4, -29.0645) -> (126, -29.0645)
  line L5 (126, -29.0645) -> (126, -68)
  line L6 (126, -68) -> (130, -67.8645)
  line L7 (130, -67.8645) -> (146.4, -67.8645)
  line L8 (146.4, -67.8645) -> (146.4, -29)
  line L9 (146.4, -29) -> (142.4, -29.0645)
  line L10 (130, -37.0645) -> (136.2, -37.0645)
  line L11 (136.2, -37.0645) -> (136.2, -34.0645)
  circle A0 centre (136.2, -34.0645) radius 1.5
  line L12 (142.4, -59.8645) -> (136.2, -59.8645)
  line L13 (136.2, -59.8645) -> (136.2, -62.8645)
  circle A1 centre (136.2, -62.8645) radius 1.5
  dimension "d174" = 6.2
  dimension "d175" = 3
  dimension "d176" = 3
  dimension "d177" = 6.2
  dimension "d178" = 3
  dimension "d179" = 3
  constraint coincident L2.end L3.start
  constraint perpendicular L0 L10
  constraint perpendicular L10 L11
  constraint coincident L11.end A0.centre
  constraint coincident L0.end L1.start
  constraint perpendicular L0 L12
  constraint perpendicular L12 L13
  constraint coincident L13.end A1.centre
  measures "d174" distance of L2.end L10.end
  measures "d175" distance of L10.end L11.end
  measures "d176" diameter of A0
  measures "d177" distance of L0.end L12.end
  measures "d178" distance of L12.end L13.end
  measures "d179" diameter of A1
extrude "Extrude38" cut sketch "Sketch25" against normal blind 20 contours A0 | A1 bodies 1
sketch "Sketch26" plane through (0, 0, 0.2628) normal (0, 0, -1) x (1, 0, 0)
  line L0 (200.2873, 0) -> (100.3336, 0)
  line L1 (100.3336, 0) -> (100.3336, -89.9645)
  line L2 (100.3336, -89.9645) -> (220.2873, -89.9645)
  line L3 (220.2873, -89.9645) -> (220.2873, 0.0355)
  line L4 (220.2873, 0.0355) -> (200.2873, 0.0355)
  line L5 (200.2873, 0.0355) -> (200.2873, 0)
  circle A0 centre (200.2873, -69.9645) radius 2.5
  circle A1 centre (120.2873, -69.9645) radius 2.5
  circle A2 centre (120.2873, -26.9645) radius 2.5
  circle A3 centre (200.2873, -26.9645) radius 2.5
  line L6 (142.4, -29.0645) -> (146.4, -29)
  line L7 (146.4, -29) -> (146.4, -67.8645)
  line L8 (146.4, -67.8645) -> (130, -67.8645)
  line L9 (130, -67.8645) -> (126, -68)
  line L10 (126, -68) -> (126, -29.0645)
  line L11 (126, -29.0645) -> (142.4, -29.0645)
  line L12 (126, -29.0645) -> (146.4, -29.0645)
  line L13 (146.4, -29.0645) -> (146.4, -67.8645)
  line L14 (146.4, -67.8645) -> (126, -67.8645)
  line L15 (126, -67.8645) -> (126, -29.0645)
  constraint horizontal L12
  constraint vertical L13
  constraint horizontal L14
  constraint vertical L15
  constraint coincident L7.end L8.start
  constraint coincident L10.end L11.start
split "Split1" by curves path "Sketch26" along L15 L12 L13 L14 bodies 1 makes body 4 at (149.007, 9.6667, 0.2628)
extrude "Extrude39" cut 1 faces at (145.0667, 29.043, -47.7372) along direction (0, 0, 1) blind 48 on bodies 4 bodies 4
extrude "Extrude40" cut 1 faces at (127.3333, 67.9097, -47.7372) along direction (0, 0, 1) blind 48 on bodies 4 bodies 4
sketch "Sketch27" plane through (0, 0, 0.2628) normal (0, 0, -1) x (1, 0, 0)
  line L0 (200.2873, 0) -> (100.3336, 0)
  line L1 (100.3336, 0) -> (100.3336, -89.9645)
  line L2 (100.3336, -89.9645) -> (220.2873, -89.9645)
  line L3 (220.2873, -89.9645) -> (220.2873, 0.0355)
  line L4 (220.2873, 0.0355) -> (200.2873, 0.0355)
  line L5 (200.2873, 0.0355) -> (200.2873, 0)
  circle A0 centre (200.2873, -69.9645) radius 2.5
  circle A1 centre (120.2873, -69.9645) radius 2.5
  circle A2 centre (120.2873, -26.9645) radius 2.5
  circle A3 centre (200.2873, -26.9645) radius 2.5
  line L6 (146.4, -29.0645) -> (146.4, -67.8645)
  line L7 (146.4, -67.8645) -> (126, -67.8645)
  line L8 (126, -67.8645) -> (126, -29.0645)
  line L9 (126, -29.0645) -> (146.4, -29.0645)
  line L10 (126, -29.0645) -> (146.4, -29.0645)
  line L11 (146.4, -29.0645) -> (146.4, -67.8645)
  line L12 (146.4, -67.8645) -> (126, -67.8645)
  line L13 (126, -67.8645) -> (126, -29.0645)
  line L14 (126, -29.0645) -> (145, -29.0645)
  line L15 (126, -29.0645) -> (136.2, -29.0645)
  line L16 (136.2, -29.0645) -> (136.2, -48.4645)
  circle A4 centre (136.2, -48.4645) radius 2
  dimension "d186" = 10.2
  dimension "d187" = 19.4
  dimension "d188" = 4
  constraint horizontal L10
  constraint vertical L11
  constraint horizontal L12
  constraint vertical L13
  constraint coincident L6.end L7.start
  constraint coincident L8.end L9.start
  constraint coincident L10 L14.end
  constraint perpendicular L13 L15
  constraint perpendicular L12 L16
  constraint coincident L16.end A4.centre
  measures "d186" distance of L8.end L15.end
  measures "d187" distance of L15.end L16.end
  measures "d188" diameter of A4
extrude "Extrude41" add sketch "Sketch27" against normal blind 7 contours L6 L7 L8 L9 L10 L11 L12 L13 L14 L15 bodies 4
extrude "Extrude42" add 1 faces at (138.2667, 52.2645, 0.2628) along direction (0, 0, -1) blind 7 on bodies 1 bodies 1
extrude "Extrude43" cut 1 faces at (139.6, 54.9311, 7.2628) along direction (0, 0, -1) blind 7 on bodies 1 bodies 1
sketch "Sketch28" plane through (0, 0, 0.2628) normal (0, 0, 1) x (-1, 0, 0)
  line L0 (-126, -67.8645) -> (-126, -29.0645)
  line L1 (-126, -29.0645) -> (-146.4, -29.0645)
  line L2 (-146.4, -29.0645) -> (-146.4, -67.8645)
  line L3 (-146.4, -67.8645) -> (-126, -67.8645)
  line L4 (-126, -50) -> (-146, -50)
  line L5 (-126, -50) -> (-136.2, -50)
  line L6 (-126, -50) -> (-136.2, -50)
  line L7 (-136.2, -50) -> (-136.2, -67.8645)
  line L8 (-136.2, -67.8645) -> (-136.2, -29.0645)
  line L9 (-136.2, -29.0645) -> (-136.2, -67.8645)
  line L10 (-136.2, -67.8645) -> (-136.2, -48.4645)
  circle A0 centre (-136.2, -48.4645) radius 2
  dimension "d195" = 10.2
  dimension "d196" = 10.2
  dimension "d197" = 19.4
  dimension "d198" = 4
  constraint horizontal L4
  constraint horizontal L5
  constraint horizontal L6
  constraint midpoint L3 L7.end
  constraint midpoint L1 L8.end
  constraint perpendicular L5 L10
  constraint coincident L10.end A0.centre
  measures "d195" distance of L4.start L5.end
  measures "d196" distance of L4.start L5.end
  measures "d197" distance of L7.end L10.end
  measures "d198" diameter of A0
sketch "Sketch29" plane through (0, 0, -6.7372) normal (0, 0, -1) x (1, 0, 0)
  line L0 (142.4, -59.3645) -> (146.4, -59.3645)
  line L1 (146.4, -59.3645) -> (146.4, -37.3645)
  line L2 (146.4, -37.3645) -> (142.4, -37.3645)
  line L3 (142.4, -37.3645) -> (142.4, -37.0645)
  line L4 (142.4, -37.0645) -> (130, -37.0645)
  line L5 (130, -37.0645) -> (130, -37.3645)
  line L6 (130, -37.3645) -> (126, -37.3645)
  line L7 (126, -37.3645) -> (126, -59.3645)
  line L8 (126, -59.3645) -> (130, -59.3645)
  line L9 (130, -59.3645) -> (130, -59.8645)
  line L10 (130, -59.8645) -> (142.4, -59.8645)
  line L11 (142.4, -59.8645) -> (142.4, -59.3645)
extrude "Extrude44" cut sketch "Sketch28" against normal blind 10 contours L4 L5 L6 L7 L8 L9 L10 A0 | L4 L5 L6 L8 L9 L10 A0 | L4 L7 L8 L9 L10 A0 | L4 L8 L9 L10 A0 bodies 1
sketch "Sketch30" plane through (0, 0, 0.2628) normal (0, 0, -1) x (1, 0, 0)
  circle A0 centre (136.2, -48.4645) radius 2
  line L0 (200.2873, 0) -> (100.3336, 0)
  line L1 (100.3336, 0) -> (100.3336, -89.9645)
  line L2 (100.3336, -89.9645) -> (220.2873, -89.9645)
  line L3 (220.2873, -89.9645) -> (220.2873, 0.0355)
  line L4 (220.2873, 0.0355) -> (200.2873, 0.0355)
  line L5 (200.2873, 0.0355) -> (200.2873, 0)
  circle A1 centre (200.2873, -69.9645) radius 2.5
  circle A2 centre (120.2873, -69.9645) radius 2.5
  circle A3 centre (120.2873, -26.9645) radius 2.5
  circle A4 centre (200.2873, -26.9645) radius 2.5
  line L6 (125, 0) -> (125, -25)
  line L7 (125, -25) -> (150.3104, -25)
  line L8 (150.3104, -25) -> (150.3104, 0)
  constraint coincident L0 L6.start
  constraint perpendicular L0 L6
  constraint perpendicular L1 L7
  constraint midpoint L0 L8.end
  constraint perpendicular L0 L8
extrude "Extrude45" cut sketch "Sketch30" against normal blind 18 contours L0 L6 L7 L8 bodies 4
extrude "Extrude46" add 1 faces at (100.3336, 59.9763, 4.9295) along direction (-1, 0, 0) blind 30 on bodies 4 bodies 4
sketch "Sketch31" plane through (0, 0, 7.2628) normal (0, 0, 1) x (-1, 0, 0)
  line L0 (-125, -25) -> (-150.2873, -25)
  line L1 (-150.2873, -25) -> (-150.2873, -69.9645)
  line L2 (-150.2873, -69.9645) -> (-155.2873, -69.9645)
  line L3 (-155.2873, -69.9645) -> (-190.2873, -69.9645)
  line L4 (-190.2873, -69.9645) -> (-190.2873, -26.9645)
  line L5 (-190.2873, -26.9645) -> (-190.2873, -21.9645)
  line L6 (-190.2873, -21.9645) -> (-150.3104, -21.9645)
  line L7 (-150.3104, -21.9645) -> (-150.3104, 0)
  line L8 (-150.3104, 0) -> (-200.2873, 0)
  line L9 (-200.2873, 0) -> (-200.2873, 0.0355)
  line L10 (-200.2873, 0.0355) -> (-220.2873, 0.0355)
  line L11 (-220.2873, 0.0355) -> (-220.2873, -89.9645)
  line L12 (-220.2873, -89.9645) -> (-70.3336, -89.9645)
  line L13 (-70.3336, -89.9645) -> (-70.3336, 0)
  line L14 (-70.3336, 0) -> (-125, 0)
  line L15 (-125, 0) -> (-125, -25)
  circle A0 centre (-136.2, -48.4645) radius 2
  circle A1 centre (-120.2873, -69.9645) radius 2.5
  circle A2 centre (-200.2873, -69.9645) radius 2.5
  circle A3 centre (-120.2873, -26.9645) radius 2.5
  circle A4 centre (-200.2873, -26.9645) radius 2.5
  line L16 (-120.2873, -26.9645) -> (-90.2873, -26.9645)
  circle A5 centre (-90.2873, -26.9645) radius 2.5
  line L17 (-120.2873, -69.9645) -> (-90.2873, -69.9645)
  circle A6 centre (-90.2873, -69.9645) radius 2.5
  dimension "d205" = 30
  dimension "d206" = 5
  dimension "d207" = 30
  dimension "d208" = 5
  constraint coincident A3.centre L16.start
  constraint perpendicular L1 L16
  constraint coincident L16.end A5.centre
  constraint coincident A1.centre L17.start
  constraint horizontal L17
  constraint coincident L17.end A6.centre
  measures "d205" distance of A3.centre L16.end
  measures "d206" diameter of A5
  measures "d207" distance of A1.centre L17.end
  measures "d208" diameter of A6
extrude "Extrude47" cut sketch "Sketch31" against normal blind 7 contours A5 | A6 bodies 4
sketch "Sketch32" plane through (0, 0, 7.2628) normal (0, 0, 1) x (-1, 0, 0)
  circle A0 centre (-90.2873, -26.9645) radius 2.5
  circle A1 centre (-90.2873, -69.9645) radius 2.5
  line L0 (-125, -25) -> (-150.2873, -25)
  line L1 (-150.2873, -25) -> (-150.2873, -69.9645)
  line L2 (-150.2873, -69.9645) -> (-155.2873, -69.9645)
  line L3 (-155.2873, -69.9645) -> (-190.2873, -69.9645)
  line L4 (-190.2873, -69.9645) -> (-190.2873, -26.9645)
  line L5 (-190.2873, -26.9645) -> (-190.2873, -21.9645)
  line L6 (-190.2873, -21.9645) -> (-150.3104, -21.9645)
  line L7 (-150.3104, -21.9645) -> (-150.3104, 0)
  line L8 (-150.3104, 0) -> (-200.2873, 0)
  line L9 (-200.2873, 0) -> (-200.2873, 0.0355)
  line L10 (-200.2873, 0.0355) -> (-220.2873, 0.0355)
  line L11 (-220.2873, 0.0355) -> (-220.2873, -89.9645)
  line L12 (-220.2873, -89.9645) -> (-70.3336, -89.9645)
  line L13 (-70.3336, -89.9645) -> (-70.3336, 0)
  line L14 (-70.3336, 0) -> (-125, 0)
  line L15 (-125, 0) -> (-125, -25)
  circle A2 centre (-136.2, -48.4645) radius 2
  circle A3 centre (-120.2873, -69.9645) radius 2.5
  circle A4 centre (-200.2873, -69.9645) radius 2.5
  circle A5 centre (-120.2873, -26.9645) radius 2.5
  circle A6 centre (-200.2873, -26.9645) radius 2.5
  circle A7 centre (-120.2873, -26.9645) radius 2.5
  circle A8 centre (-120.2873, -69.9645) radius 2.5
  constraint concentric A5 A7
  constraint concentric A3 A8
extrude "Extrude48" add sketch "Sketch32" against normal blind 7 contours A3 A8 | A5 A7 bodies 4